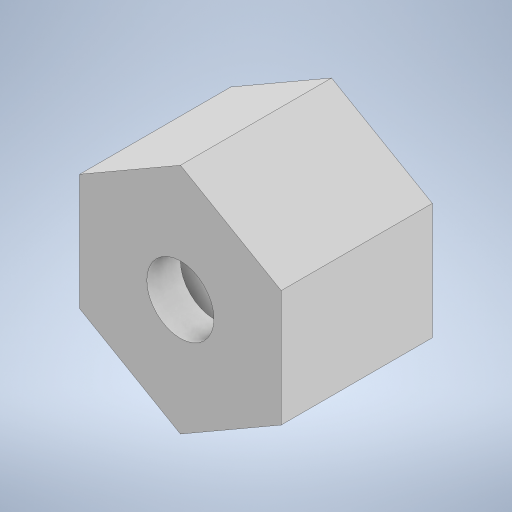
# Autodesk Inventor part: HUDSON-1-85
Saved by Autodesk Inventor 2024.2 (Build 282272000, 272)
## iProperties
Created: 2024-10-06
Part Number: HUDSON-1-85
Material: Generic
Document SubType Name: Modeling
Designer: melim
Density: 1 g/cm^3
Appearance: Default
Author: melim
Autodesk Inventor part; units mm, degrees
ref_plane "YZ Plane" through (0, 0, 0) normal (1, 0, 0) x (0, 1, 0)
ref_plane "XZ Plane" through (0, 0, 0) normal (0, 1, 0) x (-1, 0, 0)
ref_plane "XY Plane" through (0, 0, 0) normal (0, 0, 1) x (1, 0, 0)
sketch "Sketch1" plane through (0, 0, 0) normal (0, 0, 1) x (1, 0, 0)
  line L0 (0, -6.9282) -> (-6, -3.4641)
  line L1 (-6, -3.4641) -> (-6, 3.4641)
  line L2 (-6, 3.4641) -> (0, 6.9282)
  line L3 (0, 6.9282) -> (6, 3.4641)
  line L4 (6, 3.4641) -> (6, -3.4641)
  line L5 (6, -3.4641) -> (0, -6.9282)
  line L6 (0, 0) -> (0, -16.3015)
  dimension "d0" = 12
  constraints: 14 end point, 1 coincident, 1 point on line, 1 vertical, 13 other
  measures "d0" distance between parallel lines of L5 L2
extrude "Extrusion1" add sketch "Sketch1" along normal blind 9
hole "Hole1" at (0, 0, 0) direction (0, 0, 1) diameter 4 end through all counterbore diameter 8 counterbore depth 7
thread "Thread1" size "M8x1.25" class "6H" standard "ANSI Metric M Profile" full length
body "Solid1"
